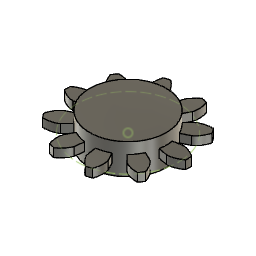
Tank Track Gear small v6 (Autodesk Fusion 360 design; units mm, degrees)
description: Spur Gear; Module: 3.0; Num Teeth: 10; Pressure Angle: 20.0; Backlash: 0.00 mm
Autodesk Fusion 360 part; units mm, degrees
(part 1 of 4)
sketch "Sketch1" plane through (0, 0, 0) normal (0, 0, 1) x (1, 0, 0) in component "Spur Gear (10 teeth)"
  circle A0 centre (0, 0) radius 11.3492
extrude "Extrude1" add sketch "Sketch1" along normal blind 2.5 in component "Spur Gear (10 teeth)"
sketch "Sketch2" plane through (0, 0, 0) normal (0, 0, 1) x (1, 0, 0) in component "Spur Gear (10 teeth)"
  spline S0 degree 5 poles (13.8874, -2.4122) (13.899, -2.4142) (13.9221, -2.4178) (13.9569, -2.422) (14.0035, -2.4254) (14.0621, -2.4264) (14.1209, -2.4253) (14.1799, -2.4228) (14.239, -2.4196) (14.2982, -2.4158) (14.3573, -2.4115) (14.4166, -2.4064) (14.4759, -2.4004) (14.5353, -2.3932) (14.5948, -2.3849) (14.6543, -2.3756) (14.7138, -2.3655) (14.7734, -2.3546) (14.8329, -2.343) (14.8925, -2.3309) (14.9521, -2.3181) (15.0117, -2.3046) (15.0713, -2.2905) (15.1308, -2.2756) (15.1904, -2.26) (15.25, -2.2438) (15.3095, -2.2269) (15.3691, -2.2094) (15.4286, -2.1913) (15.488, -2.1727) (15.5475, -2.1534) (15.6069, -2.1336) (15.6662, -2.1132) (15.7256, -2.0922) (15.7848, -2.0706) (15.8441, -2.0485) (15.9033, -2.0258) (15.9624, -2.0026) (16.0215, -1.9789) (16.0805, -1.9546) (16.1394, -1.9298) (16.1983, -1.9045) (16.2571, -1.8786) (16.3159, -1.8523) (16.3745, -1.8254) (16.4331, -1.798) (16.4917, -1.7701) (16.5501, -1.7418) (16.6085, -1.7129) (16.6667, -1.6835) (16.7249, -1.6537) (16.783, -1.6234) (16.841, -1.5926) (16.8989, -1.5613) (16.9568, -1.5296) (17.0145, -1.4974) (17.0721, -1.4647) (17.1296, -1.4316) (17.187, -1.398) (17.2443, -1.364) (17.3015, -1.3295) (17.3586, -1.2945) (17.4155, -1.2591) (17.4724, -1.2233) (17.5291, -1.187) (17.5857, -1.1503) (17.6422, -1.1132) (17.6986, -1.0756) (17.7548, -1.0376) (17.8109, -0.9992) (17.8669, -0.9603) (17.9116, -0.9289) (17.945, -0.9051) (17.9673, -0.8892) (17.9784, -0.8812) knots 0 0 0 0 0 0 0.01428571 0.02857143 0.04285714 0.05714286 0.07142857 0.08571429 0.1 0.11428571 0.12857143 0.14285714 0.15714286 0.17142857 0.18571429 0.2 0.21428571 0.22857143 0.24285714 0.25714286 0.27142857 0.28571429 0.3 0.31428571 0.32857143 0.34285714 0.35714286 0.37142857 0.38571429 0.4 0.41428571 0.42857143 0.44285714 0.45714286 0.47142857 0.48571429 0.5 0.51428571 0.52857143 0.54285714 0.55714286 0.57142857 0.58571429 0.6 0.61428571 0.62857143 0.64285714 0.65714286 0.67142857 0.68571429 0.7 0.71428571 0.72857143 0.74285714 0.75714286 0.77142857 0.78571429 0.8 0.81428571 0.82857143 0.84285714 0.85714286 0.87142857 0.88571429 0.9 0.91428571 0.92857143 0.94285714 0.95714286 0.97142857 0.98571429 1 1 1 1 1 1
  spline S1 degree 5 poles (13.8874, 2.4122) (13.899, 2.4142) (13.9221, 2.4178) (13.9569, 2.422) (14.0035, 2.4254) (14.0621, 2.4264) (14.1209, 2.4253) (14.1799, 2.4228) (14.239, 2.4196) (14.2982, 2.4158) (14.3573, 2.4115) (14.4166, 2.4064) (14.4759, 2.4004) (14.5353, 2.3932) (14.5948, 2.3849) (14.6543, 2.3756) (14.7138, 2.3655) (14.7734, 2.3546) (14.8329, 2.343) (14.8925, 2.3309) (14.9521, 2.3181) (15.0117, 2.3046) (15.0713, 2.2905) (15.1308, 2.2756) (15.1904, 2.26) (15.25, 2.2438) (15.3095, 2.2269) (15.3691, 2.2094) (15.4286, 2.1913) (15.488, 2.1727) (15.5475, 2.1534) (15.6069, 2.1336) (15.6662, 2.1132) (15.7256, 2.0922) (15.7848, 2.0706) (15.8441, 2.0485) (15.9033, 2.0258) (15.9624, 2.0026) (16.0215, 1.9789) (16.0805, 1.9546) (16.1394, 1.9298) (16.1983, 1.9045) (16.2571, 1.8786) (16.3159, 1.8523) (16.3745, 1.8254) (16.4331, 1.798) (16.4917, 1.7701) (16.5501, 1.7418) (16.6085, 1.7129) (16.6667, 1.6835) (16.7249, 1.6537) (16.783, 1.6234) (16.841, 1.5926) (16.8989, 1.5613) (16.9568, 1.5296) (17.0145, 1.4974) (17.0721, 1.4647) (17.1296, 1.4316) (17.187, 1.398) (17.2443, 1.364) (17.3015, 1.3295) (17.3586, 1.2945) (17.4155, 1.2591) (17.4724, 1.2233) (17.5291, 1.187) (17.5857, 1.1503) (17.6422, 1.1132) (17.6986, 1.0756) (17.7548, 1.0376) (17.8109, 0.9992) (17.8669, 0.9603) (17.9116, 0.9289) (17.945, 0.9051) (17.9673, 0.8892) (17.9784, 0.8812) knots 0 0 0 0 0 0 0.01428571 0.02857143 0.04285714 0.05714286 0.07142857 0.08571429 0.1 0.11428571 0.12857143 0.14285714 0.15714286 0.17142857 0.18571429 0.2 0.21428571 0.22857143 0.24285714 0.25714286 0.27142857 0.28571429 0.3 0.31428571 0.32857143 0.34285714 0.35714286 0.37142857 0.38571429 0.4 0.41428571 0.42857143 0.44285714 0.45714286 0.47142857 0.48571429 0.5 0.51428571 0.52857143 0.54285714 0.55714286 0.57142857 0.58571429 0.6 0.61428571 0.62857143 0.64285714 0.65714286 0.67142857 0.68571429 0.7 0.71428571 0.72857143 0.74285714 0.75714286 0.77142857 0.78571429 0.8 0.81428571 0.82857143 0.84285714 0.85714286 0.87142857 0.88571429 0.9 0.91428571 0.92857143 0.94285714 0.95714286 0.97142857 0.98571429 1 1 1 1 1 1
  arc A0 (17.9784, -0.8812) -> (17.9784, 0.8812) centre (0, 0) ccw
  line L0 (11.1719, -1.9423) -> (13.8874, -2.4122)
  line L1 (11.1719, 1.9423) -> (13.8874, 2.4122)
  line L2 (11.1719, -1.9423) -> (11.1719, 1.9423)
  point P0 (14.1686, -2.4231)
  point P1 (14.4549, -2.4023)
  point P2 (14.7445, -2.3598)
  point P3 (15.0363, -2.2987)
  point P4 (15.3299, -2.2208)
  point P5 (15.6246, -2.1274)
  point P6 (15.9202, -2.0191)
  point P7 (16.2161, -1.8966)
  point P8 (16.5119, -1.7602)
  point P9 (16.8074, -1.6104)
  point P10 (17.1022, -1.4473)
  point P11 (17.3958, -1.2713)
  point P12 (17.688, -1.0826)
  point P13 (14.1686, 2.4231)
  point P14 (14.4549, 2.4023)
  point P15 (14.7445, 2.3598)
  point P16 (15.0363, 2.2987)
  point P17 (15.3299, 2.2208)
  point P18 (15.6246, 2.1274)
  point P19 (15.9202, 2.0191)
  point P20 (16.2161, 1.8966)
  point P21 (16.5119, 1.7602)
  point P22 (16.8074, 1.6104)
  point P23 (17.1022, 1.4473)
  point P24 (17.3958, 1.2713)
  point P25 (17.688, 1.0826)
extrude "Extrude2" add sketch "Sketch2" along normal blind 2.5 in component "Spur Gear (10 teeth)"
pattern_circular "C-Pattern1" count 10 over 360 about axis through (0, 0, 0) along (0, 0, 1) of "Extrude2" in component "Spur Gear (10 teeth)"
sketch "Sketch3" plane through (0, 0, 0) normal (0, 0, 1) x (1, 0, 0) in component "Spur Gear (10 teeth)"
  circle A0 centre (0, 0) radius 15 construction
sketch "Sketch1 (2)" plane through (0, 0, 2.5) normal (0, 0, 1) x (-1, 0, 0)
  arc A0 (-10.1886, 4.9996) -> (-11.1815, 1.9439) centre (0, 0) ccw
  line L0 (-11.1815, 1.9439) -> (-13.8874, 2.4122)
  spline S0 degree 5 poles (-13.8874, 2.4122) (-13.899, 2.4142) (-13.9221, 2.4178) (-13.9569, 2.422) (-14.0035, 2.4254) (-14.0621, 2.4264) (-14.1209, 2.4253) (-14.1799, 2.4228) (-14.239, 2.4196) (-14.2982, 2.4158) (-14.3573, 2.4115) (-14.4166, 2.4064) (-14.4759, 2.4004) (-14.5353, 2.3932) (-14.5948, 2.3849) (-14.6543, 2.3756) (-14.7138, 2.3655) (-14.7734, 2.3546) (-14.8329, 2.343) (-14.8925, 2.3309) (-14.9521, 2.3181) (-15.0117, 2.3046) (-15.0713, 2.2905) (-15.1308, 2.2756) (-15.1904, 2.26) (-15.25, 2.2438) (-15.3095, 2.2269) (-15.3691, 2.2094) (-15.4286, 2.1913) (-15.488, 2.1727) (-15.5475, 2.1534) (-15.6069, 2.1336) (-15.6662, 2.1132) (-15.7256, 2.0922) (-15.7848, 2.0706) (-15.8441, 2.0485) (-15.9033, 2.0258) (-15.9624, 2.0026) (-16.0215, 1.9789) (-16.0805, 1.9546) (-16.1394, 1.9298) (-16.1983, 1.9045) (-16.2571, 1.8786) (-16.3159, 1.8523) (-16.3745, 1.8254) (-16.4331, 1.798) (-16.4917, 1.7701) (-16.5501, 1.7418) (-16.6085, 1.7129) (-16.6667, 1.6835) (-16.7249, 1.6537) (-16.783, 1.6234) (-16.841, 1.5926) (-16.8989, 1.5613) (-16.9568, 1.5296) (-17.0145, 1.4974) (-17.0721, 1.4647) (-17.1296, 1.4316) (-17.187, 1.398) (-17.2443, 1.364) (-17.3015, 1.3295) (-17.3586, 1.2945) (-17.4155, 1.2591) (-17.4724, 1.2233) (-17.5291, 1.187) (-17.5857, 1.1503) (-17.6422, 1.1132) (-17.6986, 1.0756) (-17.7548, 1.0376) (-17.8109, 0.9992) (-17.8669, 0.9603) (-17.9116, 0.9289) (-17.945, 0.9051) (-17.9673, 0.8892) (-17.9784, 0.8812) knots 0 0 0 0 0 0 0.01428571 0.02857143 0.04285714 0.05714286 0.07142857 0.08571429 0.1 0.11428571 0.12857143 0.14285714 0.15714286 0.17142857 0.18571429 0.2 0.21428571 0.22857143 0.24285714 0.25714286 0.27142857 0.28571429 0.3 0.31428571 0.32857143 0.34285714 0.35714286 0.37142857 0.38571429 0.4 0.41428571 0.42857143 0.44285714 0.45714286 0.47142857 0.48571429 0.5 0.51428571 0.52857143 0.54285714 0.55714286 0.57142857 0.58571429 0.6 0.61428571 0.62857143 0.64285714 0.65714286 0.67142857 0.68571429 0.7 0.71428571 0.72857143 0.74285714 0.75714286 0.77142857 0.78571429 0.8 0.81428571 0.82857143 0.84285714 0.85714286 0.87142857 0.88571429 0.9 0.91428571 0.92857143 0.94285714 0.95714286 0.97142857 0.98571429 1 1 1 1 1 1
  arc A1 (-17.9784, 0.8812) -> (-17.9784, -0.8812) centre (0, 0) ccw
  spline S1 degree 5 poles (-17.9784, -0.8812) (-17.9673, -0.8892) (-17.945, -0.9051) (-17.9116, -0.9289) (-17.8669, -0.9603) (-17.8109, -0.9992) (-17.7548, -1.0376) (-17.6986, -1.0756) (-17.6422, -1.1132) (-17.5857, -1.1503) (-17.5291, -1.187) (-17.4724, -1.2233) (-17.4155, -1.2591) (-17.3586, -1.2945) (-17.3015, -1.3295) (-17.2443, -1.364) (-17.187, -1.398) (-17.1296, -1.4316) (-17.0721, -1.4647) (-17.0145, -1.4974) (-16.9568, -1.5296) (-16.8989, -1.5613) (-16.841, -1.5926) (-16.783, -1.6234) (-16.7249, -1.6537) (-16.6667, -1.6835) (-16.6085, -1.7129) (-16.5501, -1.7418) (-16.4917, -1.7701) (-16.4331, -1.798) (-16.3745, -1.8254) (-16.3159, -1.8523) (-16.2571, -1.8786) (-16.1983, -1.9045) (-16.1394, -1.9298) (-16.0805, -1.9546) (-16.0215, -1.9789) (-15.9624, -2.0026) (-15.9033, -2.0258) (-15.8441, -2.0485) (-15.7848, -2.0706) (-15.7256, -2.0922) (-15.6662, -2.1132) (-15.6069, -2.1336) (-15.5475, -2.1534) (-15.488, -2.1727) (-15.4286, -2.1913) (-15.3691, -2.2094) (-15.3095, -2.2269) (-15.25, -2.2438) (-15.1904, -2.26) (-15.1308, -2.2756) (-15.0713, -2.2905) (-15.0117, -2.3046) (-14.9521, -2.3181) (-14.8925, -2.3309) (-14.8329, -2.343) (-14.7734, -2.3546) (-14.7138, -2.3655) (-14.6543, -2.3756) (-14.5948, -2.3849) (-14.5353, -2.3932) (-14.4759, -2.4004) (-14.4166, -2.4064) (-14.3573, -2.4115) (-14.2982, -2.4158) (-14.239, -2.4196) (-14.1799, -2.4228) (-14.1209, -2.4253) (-14.0621, -2.4264) (-14.0035, -2.4254) (-13.9569, -2.422) (-13.9221, -2.4178) (-13.899, -2.4142) (-13.8874, -2.4122) knots -1 -1 -1 -1 -1 -1 -0.98571429 -0.97142857 -0.95714286 -0.94285714 -0.92857143 -0.91428571 -0.9 -0.88571429 -0.87142857 -0.85714286 -0.84285714 -0.82857143 -0.81428571 -0.8 -0.78571429 -0.77142857 -0.75714286 -0.74285714 -0.72857143 -0.71428571 -0.7 -0.68571429 -0.67142857 -0.65714286 -0.64285714 -0.62857143 -0.61428571 -0.6 -0.58571429 -0.57142857 -0.55714286 -0.54285714 -0.52857143 -0.51428571 -0.5 -0.48571429 -0.47142857 -0.45714286 -0.44285714 -0.42857143 -0.41428571 -0.4 -0.38571429 -0.37142857 -0.35714286 -0.34285714 -0.32857143 -0.31428571 -0.3 -0.28571429 -0.27142857 -0.25714286 -0.24285714 -0.22857143 -0.21428571 -0.2 -0.18571429 -0.17142857 -0.15714286 -0.14285714 -0.12857143 -0.11428571 -0.1 -0.08571429 -0.07142857 -0.05714286 -0.04285714 -0.02857143 -0.01428571 0 0 0 0 0 0
  line L1 (-13.8874, -2.4122) -> (-11.1815, -1.9439)
  arc A2 (-11.1815, -1.9439) -> (-10.1886, -4.9996) centre (0, 0) ccw
  line L2 (-10.1886, -4.9996) -> (-12.6531, -6.2113)
  spline S2 degree 5 poles (-12.6531, -6.2113) (-12.6636, -6.2165) (-12.6844, -6.2271) (-12.715, -6.2442) (-12.7547, -6.2689) (-12.8027, -6.3025) (-12.8496, -6.338) (-12.8959, -6.3747) (-12.9418, -6.412) (-12.9874, -6.4498) (-13.0328, -6.4881) (-13.0777, -6.527) (-13.1222, -6.5668) (-13.166, -6.6075) (-13.2092, -6.6491) (-13.2519, -6.6916) (-13.2941, -6.7349) (-13.3359, -6.7787) (-13.3773, -6.823) (-13.4183, -6.8679) (-13.459, -6.9133) (-13.4993, -6.9592) (-13.5392, -7.0056) (-13.5787, -7.0527) (-13.6177, -7.1003) (-13.6564, -7.1485) (-13.6946, -7.1971) (-13.7325, -7.2463) (-13.77, -7.2959) (-13.8071, -7.3459) (-13.8439, -7.3964) (-13.8803, -7.4474) (-13.9163, -7.4988) (-13.952, -7.5506) (-13.9873, -7.6029) (-14.0222, -7.6556) (-14.0568, -7.7088) (-14.091, -7.7623) (-14.1248, -7.8162) (-14.1583, -7.8706) (-14.1914, -7.9253) (-14.2241, -7.9804) (-14.2565, -8.0359) (-14.2885, -8.0917) (-14.3202, -8.1479) (-14.3515, -8.2045) (-14.3825, -8.2615) (-14.4131, -8.3188) (-14.4433, -8.3764) (-14.4732, -8.4344) (-14.5028, -8.4928) (-14.532, -8.5515) (-14.5608, -8.6105) (-14.5893, -8.6698) (-14.6174, -8.7295) (-14.6451, -8.7894) (-14.6726, -8.8497) (-14.6996, -8.9103) (-14.7263, -8.9713) (-14.7527, -9.0325) (-14.7786, -9.094) (-14.8043, -9.1558) (-14.8296, -9.2179) (-14.8545, -9.2803) (-14.8791, -9.343) (-14.9033, -9.406) (-14.9272, -9.4692) (-14.9507, -9.5328) (-14.9738, -9.5966) (-14.9966, -9.6606) (-15.0191, -9.725) (-15.0367, -9.7767) (-15.0498, -9.8156) (-15.0585, -9.8415) (-15.0628, -9.8545) knots 0 0 0 0 0 0 0.01428571 0.02857143 0.04285714 0.05714286 0.07142857 0.08571429 0.1 0.11428571 0.12857143 0.14285714 0.15714286 0.17142857 0.18571429 0.2 0.21428571 0.22857143 0.24285714 0.25714286 0.27142857 0.28571429 0.3 0.31428571 0.32857143 0.34285714 0.35714286 0.37142857 0.38571429 0.4 0.41428571 0.42857143 0.44285714 0.45714286 0.47142857 0.48571429 0.5 0.51428571 0.52857143 0.54285714 0.55714286 0.57142857 0.58571429 0.6 0.61428571 0.62857143 0.64285714 0.65714286 0.67142857 0.68571429 0.7 0.71428571 0.72857143 0.74285714 0.75714286 0.77142857 0.78571429 0.8 0.81428571 0.82857143 0.84285714 0.85714286 0.87142857 0.88571429 0.9 0.91428571 0.92857143 0.94285714 0.95714286 0.97142857 0.98571429 1 1 1 1 1 1
  arc A3 (-15.0628, -9.8545) -> (-14.0269, -11.2804) centre (0, 0) ccw
  spline S3 degree 5 poles (-14.0269, -11.2804) (-14.0132, -11.2803) (-13.9858, -11.2801) (-13.9448, -11.2796) (-13.8902, -11.2788) (-13.822, -11.2773) (-13.754, -11.2754) (-13.6862, -11.2731) (-13.6185, -11.2704) (-13.551, -11.2673) (-13.4836, -11.2637) (-13.4164, -11.2597) (-13.3494, -11.2553) (-13.2825, -11.2504) (-13.2158, -11.2451) (-13.1492, -11.2394) (-13.0829, -11.2333) (-13.0167, -11.2267) (-12.9507, -11.2197) (-12.8849, -11.2123) (-12.8192, -11.2044) (-12.7538, -11.1961) (-12.6886, -11.1873) (-12.6235, -11.1782) (-12.5587, -11.1685) (-12.4941, -11.1585) (-12.4297, -11.148) (-12.3655, -11.137) (-12.3016, -11.1256) (-12.2378, -11.1138) (-12.1743, -11.1015) (-12.1111, -11.0887) (-12.0481, -11.0755) (-11.9853, -11.0619) (-11.9228, -11.0477) (-11.8605, -11.0332) (-11.7985, -11.0181) (-11.7367, -11.0026) (-11.6752, -10.9866) (-11.614, -10.9702) (-11.5531, -10.9533) (-11.4925, -10.9359) (-11.4322, -10.918) (-11.3721, -10.8996) (-11.3124, -10.8807) (-11.253, -10.8614) (-11.1939, -10.8415) (-11.1352, -10.8212) (-11.0767, -10.8003) (-11.0186, -10.779) (-10.9609, -10.7571) (-10.9036, -10.7347) (-10.8466, -10.7117) (-10.7901, -10.6881) (-10.734, -10.664) (-10.6782, -10.6393) (-10.6229, -10.6141) (-10.5679, -10.5884) (-10.5133, -10.5623) (-10.4592, -10.5355) (-10.4056, -10.508) (-10.3526, -10.4798) (-10.3004, -10.4507) (-10.2488, -10.4207) (-10.1979, -10.39) (-10.1475, -10.3587) (-10.0974, -10.3269) (-10.0477, -10.2948) (-9.9985, -10.2622) (-9.9503, -10.2285) (-9.9035, -10.1932) (-9.8677, -10.1631) (-9.842, -10.1393) (-9.8255, -10.1228) (-9.8173, -10.1144) knots -1 -1 -1 -1 -1 -1 -0.98571429 -0.97142857 -0.95714286 -0.94285714 -0.92857143 -0.91428571 -0.9 -0.88571429 -0.87142857 -0.85714286 -0.84285714 -0.82857143 -0.81428571 -0.8 -0.78571429 -0.77142857 -0.75714286 -0.74285714 -0.72857143 -0.71428571 -0.7 -0.68571429 -0.67142857 -0.65714286 -0.64285714 -0.62857143 -0.61428571 -0.6 -0.58571429 -0.57142857 -0.55714286 -0.54285714 -0.52857143 -0.51428571 -0.5 -0.48571429 -0.47142857 -0.45714286 -0.44285714 -0.42857143 -0.41428571 -0.4 -0.38571429 -0.37142857 -0.35714286 -0.34285714 -0.32857143 -0.31428571 -0.3 -0.28571429 -0.27142857 -0.25714286 -0.24285714 -0.22857143 -0.21428571 -0.2 -0.18571429 -0.17142857 -0.15714286 -0.14285714 -0.12857143 -0.11428571 -0.1 -0.08571429 -0.07142857 -0.05714286 -0.04285714 -0.02857143 -0.01428571 0 0 0 0 0 0
  line L3 (-9.8173, -10.1144) -> (-7.9034, -8.145)
  arc A4 (-7.9034, -8.145) -> (-5.3041, -10.0335) centre (0, 0) ccw
  line L4 (-5.3041, -10.0335) -> (-6.5856, -12.4623)
  spline S4 degree 5 poles (-6.5856, -12.4623) (-6.5911, -12.4727) (-6.6017, -12.4936) (-6.6164, -12.5253) (-6.634, -12.5687) (-6.6531, -12.6241) (-6.6702, -12.6804) (-6.6861, -12.7372) (-6.7012, -12.7944) (-6.7159, -12.8518) (-6.7301, -12.9095) (-6.7436, -12.9674) (-6.7562, -13.0257) (-6.7677, -13.0844) (-6.7782, -13.1435) (-6.7878, -13.2029) (-6.7965, -13.2627) (-6.8045, -13.3227) (-6.812, -13.3829) (-6.8188, -13.4433) (-6.8251, -13.504) (-6.8307, -13.5648) (-6.8356, -13.6258) (-6.8399, -13.6871) (-6.8435, -13.7486) (-6.8465, -13.8102) (-6.8488, -13.8721) (-6.8506, -13.9341) (-6.8518, -13.9963) (-6.8524, -14.0586) (-6.8524, -14.1211) (-6.852, -14.1837) (-6.8509, -14.2465) (-6.8493, -14.3094) (-6.8471, -14.3724) (-6.8443, -14.4356) (-6.8411, -14.4989) (-6.8373, -14.5623) (-6.8329, -14.6258) (-6.8281, -14.6894) (-6.8227, -14.7532) (-6.8168, -14.817) (-6.8104, -14.8809) (-6.8035, -14.9449) (-6.7961, -15.009) (-6.7881, -15.0732) (-6.7797, -15.1375) (-6.7708, -15.2019) (-6.7614, -15.2663) (-6.7515, -15.3308) (-6.7411, -15.3953) (-6.7302, -15.4599) (-6.7188, -15.5246) (-6.707, -15.5894) (-6.6947, -15.6542) (-6.6819, -15.719) (-6.6686, -15.7839) (-6.6549, -15.8488) (-6.6407, -15.9138) (-6.626, -15.9788) (-6.6109, -16.0439) (-6.5953, -16.109) (-6.5792, -16.1741) (-6.5627, -16.2392) (-6.5457, -16.3044) (-6.5283, -16.3695) (-6.5104, -16.4347) (-6.4921, -16.5) (-6.4734, -16.5652) (-6.4541, -16.6304) (-6.4345, -16.6957) (-6.4184, -16.7479) (-6.4061, -16.787) (-6.3979, -16.8131) (-6.3937, -16.8262) knots 0 0 0 0 0 0 0.01428571 0.02857143 0.04285714 0.05714286 0.07142857 0.08571429 0.1 0.11428571 0.12857143 0.14285714 0.15714286 0.17142857 0.18571429 0.2 0.21428571 0.22857143 0.24285714 0.25714286 0.27142857 0.28571429 0.3 0.31428571 0.32857143 0.34285714 0.35714286 0.37142857 0.38571429 0.4 0.41428571 0.42857143 0.44285714 0.45714286 0.47142857 0.48571429 0.5 0.51428571 0.52857143 0.54285714 0.55714286 0.57142857 0.58571429 0.6 0.61428571 0.62857143 0.64285714 0.65714286 0.67142857 0.68571429 0.7 0.71428571 0.72857143 0.74285714 0.75714286 0.77142857 0.78571429 0.8 0.81428571 0.82857143 0.84285714 0.85714286 0.87142857 0.88571429 0.9 0.91428571 0.92857143 0.94285714 0.95714286 0.97142857 0.98571429 1 1 1 1 1 1
  arc A5 (-6.3937, -16.8262) -> (-4.7175, -17.3708) centre (0, 0) ccw
  spline S5 degree 5 poles (-4.7175, -17.3708) (-4.7065, -17.3627) (-4.6845, -17.3464) (-4.6516, -17.3219) (-4.6079, -17.2892) (-4.5536, -17.2479) (-4.4997, -17.2065) (-4.4462, -17.1647) (-4.393, -17.1227) (-4.3403, -17.0805) (-4.2879, -17.038) (-4.2358, -16.9952) (-4.1842, -16.9523) (-4.1329, -16.909) (-4.0821, -16.8655) (-4.0316, -16.8218) (-3.9815, -16.7778) (-3.9318, -16.7336) (-3.8825, -16.6891) (-3.8337, -16.6444) (-3.7852, -16.5995) (-3.7371, -16.5543) (-3.6895, -16.5089) (-3.6423, -16.4633) (-3.5955, -16.4174) (-3.5492, -16.3713) (-3.5032, -16.3249) (-3.4578, -16.2783) (-3.4127, -16.2315) (-3.3681, -16.1845) (-3.324, -16.1372) (-3.2803, -16.0897) (-3.2371, -16.042) (-3.1943, -15.994) (-3.152, -15.9458) (-3.1102, -15.8974) (-3.0689, -15.8488) (-3.028, -15.8) (-2.9877, -15.7509) (-2.9478, -15.7016) (-2.9085, -15.6521) (-2.8697, -15.6024) (-2.8314, -15.5525) (-2.7936, -15.5023) (-2.7564, -15.452) (-2.7197, -15.4014) (-2.6836, -15.3506) (-2.648, -15.2996) (-2.613, -15.2484) (-2.5785, -15.197) (-2.5447, -15.1453) (-2.5115, -15.0935) (-2.4789, -15.0414) (-2.447, -14.9891) (-2.4158, -14.9366) (-2.3853, -14.8839) (-2.3553, -14.831) (-2.3259, -14.7779) (-2.2971, -14.7246) (-2.2691, -14.6711) (-2.2418, -14.6174) (-2.2156, -14.5634) (-2.1904, -14.5092) (-2.1664, -14.4546) (-2.1432, -14.3998) (-2.1208, -14.3449) (-2.099, -14.2898) (-2.0776, -14.2346) (-2.057, -14.1793) (-2.0378, -14.1237) (-2.0207, -14.0676) (-2.0094, -14.0223) (-2.0027, -13.9879) (-1.9989, -13.9648) (-1.9973, -13.9532) knots -1 -1 -1 -1 -1 -1 -0.98571429 -0.97142857 -0.95714286 -0.94285714 -0.92857143 -0.91428571 -0.9 -0.88571429 -0.87142857 -0.85714286 -0.84285714 -0.82857143 -0.81428571 -0.8 -0.78571429 -0.77142857 -0.75714286 -0.74285714 -0.72857143 -0.71428571 -0.7 -0.68571429 -0.67142857 -0.65714286 -0.64285714 -0.62857143 -0.61428571 -0.6 -0.58571429 -0.57142857 -0.55714286 -0.54285714 -0.52857143 -0.51428571 -0.5 -0.48571429 -0.47142857 -0.45714286 -0.44285714 -0.42857143 -0.41428571 -0.4 -0.38571429 -0.37142857 -0.35714286 -0.34285714 -0.32857143 -0.31428571 -0.3 -0.28571429 -0.27142857 -0.25714286 -0.24285714 -0.22857143 -0.21428571 -0.2 -0.18571429 -0.17142857 -0.15714286 -0.14285714 -0.12857143 -0.11428571 -0.1 -0.08571429 -0.07142857 -0.05714286 -0.04285714 -0.02857143 -0.01428571 0 0 0 0 0 0
  line L5 (-1.9973, -13.9532) -> (-1.6065, -11.2349)
  arc A6 (-1.6065, -11.2349) -> (1.6065, -11.2349) centre (0, 0) ccw
  line L6 (1.6065, -11.2349) -> (1.9973, -13.9532)
  spline S6 degree 5 poles (1.9973, -13.9532) (1.9989, -13.9648) (2.0027, -13.9879) (2.0094, -14.0223) (2.0207, -14.0676) (2.0378, -14.1237) (2.057, -14.1793) (2.0776, -14.2346) (2.099, -14.2898) (2.1208, -14.3449) (2.1432, -14.3998) (2.1664, -14.4546) (2.1904, -14.5092) (2.2156, -14.5634) (2.2418, -14.6174) (2.2691, -14.6711) (2.2971, -14.7246) (2.3259, -14.7779) (2.3553, -14.831) (2.3853, -14.8839) (2.4158, -14.9366) (2.447, -14.9891) (2.4789, -15.0414) (2.5115, -15.0935) (2.5447, -15.1453) (2.5785, -15.197) (2.613, -15.2484) (2.648, -15.2996) (2.6836, -15.3506) (2.7197, -15.4014) (2.7564, -15.452) (2.7936, -15.5023) (2.8314, -15.5525) (2.8697, -15.6024) (2.9085, -15.6521) (2.9478, -15.7016) (2.9877, -15.7509) (3.028, -15.8) (3.0689, -15.8488) (3.1102, -15.8974) (3.152, -15.9458) (3.1943, -15.994) (3.2371, -16.042) (3.2803, -16.0897) (3.324, -16.1372) (3.3681, -16.1845) (3.4127, -16.2315) (3.4578, -16.2783) (3.5032, -16.3249) (3.5492, -16.3713) (3.5955, -16.4174) (3.6423, -16.4633) (3.6895, -16.5089) (3.7371, -16.5543) (3.7852, -16.5995) (3.8337, -16.6444) (3.8825, -16.6891) (3.9318, -16.7336) (3.9815, -16.7778) (4.0316, -16.8218) (4.0821, -16.8655) (4.1329, -16.909) (4.1842, -16.9523) (4.2358, -16.9952) (4.2879, -17.038) (4.3403, -17.0805) (4.393, -17.1227) (4.4462, -17.1647) (4.4997, -17.2065) (4.5536, -17.2479) (4.6079, -17.2892) (4.6516, -17.3219) (4.6845, -17.3464) (4.7065, -17.3627) (4.7175, -17.3708) knots 0 0 0 0 0 0 0.01428571 0.02857143 0.04285714 0.05714286 0.07142857 0.08571429 0.1 0.11428571 0.12857143 0.14285714 0.15714286 0.17142857 0.18571429 0.2 0.21428571 0.22857143 0.24285714 0.25714286 0.27142857 0.28571429 0.3 0.31428571 0.32857143 0.34285714 0.35714286 0.37142857 0.38571429 0.4 0.41428571 0.42857143 0.44285714 0.45714286 0.47142857 0.48571429 0.5 0.51428571 0.52857143 0.54285714 0.55714286 0.57142857 0.58571429 0.6 0.61428571 0.62857143 0.64285714 0.65714286 0.67142857 0.68571429 0.7 0.71428571 0.72857143 0.74285714 0.75714286 0.77142857 0.78571429 0.8 0.81428571 0.82857143 0.84285714 0.85714286 0.87142857 0.88571429 0.9 0.91428571 0.92857143 0.94285714 0.95714286 0.97142857 0.98571429 1 1 1 1 1 1
  arc A7 (4.7175, -17.3708) -> (6.3937, -16.8262) centre (0, 0) ccw
  spline S7 degree 5 poles (6.3937, -16.8262) (6.3979, -16.8131) (6.4061, -16.787) (6.4184, -16.7479) (6.4345, -16.6957) (6.4541, -16.6304) (6.4734, -16.5652) (6.4921, -16.5) (6.5104, -16.4347) (6.5283, -16.3695) (6.5457, -16.3044) (6.5627, -16.2392) (6.5792, -16.1741) (6.5953, -16.109) (6.6109, -16.0439) (6.626, -15.9788) (6.6407, -15.9138) (6.6549, -15.8488) (6.6686, -15.7839) (6.6819, -15.719) (6.6947, -15.6542) (6.707, -15.5894) (6.7188, -15.5246) (6.7302, -15.4599) (6.7411, -15.3953) (6.7515, -15.3308) (6.7614, -15.2663) (6.7708, -15.2019) (6.7797, -15.1375) (6.7881, -15.0732) (6.7961, -15.009) (6.8035, -14.9449) (6.8104, -14.8809) (6.8168, -14.817) (6.8227, -14.7532) (6.8281, -14.6894) (6.8329, -14.6258) (6.8373, -14.5623) (6.8411, -14.4989) (6.8443, -14.4356) (6.8471, -14.3724) (6.8493, -14.3094) (6.8509, -14.2465) (6.852, -14.1837) (6.8524, -14.1211) (6.8524, -14.0586) (6.8518, -13.9963) (6.8506, -13.9341) (6.8488, -13.8721) (6.8465, -13.8102) (6.8435, -13.7486) (6.8399, -13.6871) (6.8356, -13.6258) (6.8307, -13.5648) (6.8251, -13.504) (6.8188, -13.4433) (6.812, -13.3829) (6.8045, -13.3227) (6.7965, -13.2627) (6.7878, -13.2029) (6.7782, -13.1435) (6.7677, -13.0844) (6.7562, -13.0257) (6.7436, -12.9674) (6.7301, -12.9095) (6.7159, -12.8518) (6.7012, -12.7944) (6.6861, -12.7372) (6.6702, -12.6804) (6.6531, -12.6241) (6.634, -12.5687) (6.6164, -12.5253) (6.6017, -12.4936) (6.5911, -12.4727) (6.5856, -12.4623) knots -1 -1 -1 -1 -1 -1 -0.98571429 -0.97142857 -0.95714286 -0.94285714 -0.92857143 -0.91428571 -0.9 -0.88571429 -0.87142857 -0.85714286 -0.84285714 -0.82857143 -0.81428571 -0.8 -0.78571429 -0.77142857 -0.75714286 -0.74285714 -0.72857143 -0.71428571 -0.7 -0.68571429 -0.67142857 -0.65714286 -0.64285714 -0.62857143 -0.61428571 -0.6 -0.58571429 -0.57142857 -0.55714286 -0.54285714 -0.52857143 -0.51428571 -0.5 -0.48571429 -0.47142857 -0.45714286 -0.44285714 -0.42857143 -0.41428571 -0.4 -0.38571429 -0.37142857 -0.35714286 -0.34285714 -0.32857143 -0.31428571 -0.3 -0.28571429 -0.27142857 -0.25714286 -0.24285714 -0.22857143 -0.21428571 -0.2 -0.18571429 -0.17142857 -0.15714286 -0.14285714 -0.12857143 -0.11428571 -0.1 -0.08571429 -0.07142857 -0.05714286 -0.04285714 -0.02857143 -0.01428571 0 0 0 0 0 0
  line L7 (6.5856, -12.4623) -> (5.3041, -10.0335)
  arc A8 (5.3041, -10.0335) -> (7.9034, -8.145) centre (0, 0) ccw
  line L8 (7.9034, -8.145) -> (9.8173, -10.1144)
  spline S8 degree 5 poles (9.8173, -10.1144) (9.8255, -10.1228) (9.842, -10.1393) (9.8677, -10.1631) (9.9035, -10.1932) (9.9503, -10.2285) (9.9985, -10.2622) (10.0477, -10.2948) (10.0974, -10.3269) (10.1475, -10.3587) (10.1979, -10.39) (10.2488, -10.4207) (10.3004, -10.4507) (10.3526, -10.4798) (10.4056, -10.508) (10.4592, -10.5355) (10.5133, -10.5623) (10.5679, -10.5884) (10.6229, -10.6141) (10.6782, -10.6393) (10.734, -10.664) (10.7901, -10.6881) (10.8466, -10.7117) (10.9036, -10.7347) (10.9609, -10.7571) (11.0186, -10.779) (11.0767, -10.8003) (11.1352, -10.8212) (11.1939, -10.8415) (11.253, -10.8614) (11.3124, -10.8807) (11.3721, -10.8996) (11.4322, -10.918) (11.4925, -10.9359) (11.5531, -10.9533) (11.614, -10.9702) (11.6752, -10.9866) (11.7367, -11.0026) (11.7985, -11.0181) (11.8605, -11.0332) (11.9228, -11.0477) (11.9853, -11.0619) (12.0481, -11.0755) (12.1111, -11.0887) (12.1743, -11.1015) (12.2378, -11.1138) (12.3016, -11.1256) (12.3655, -11.137) (12.4297, -11.148) (12.4941, -11.1585) (12.5587, -11.1685) (12.6235, -11.1782) (12.6886, -11.1873) (12.7538, -11.1961) (12.8192, -11.2044) (12.8849, -11.2123) (12.9507, -11.2197) (13.0167, -11.2267) (13.0829, -11.2333) (13.1492, -11.2394) (13.2158, -11.2451) (13.2825, -11.2504) (13.3494, -11.2553) (13.4164, -11.2597) (13.4836, -11.2637) (13.551, -11.2673) (13.6185, -11.2704) (13.6862, -11.2731) (13.754, -11.2754) (13.822, -11.2773) (13.8902, -11.2788) (13.9448, -11.2796) (13.9858, -11.2801) (14.0132, -11.2803) (14.0269, -11.2804) knots 0 0 0 0 0 0 0.01428571 0.02857143 0.04285714 0.05714286 0.07142857 0.08571429 0.1 0.11428571 0.12857143 0.14285714 0.15714286 0.17142857 0.18571429 0.2 0.21428571 0.22857143 0.24285714 0.25714286 0.27142857 0.28571429 0.3 0.31428571 0.32857143 0.34285714 0.35714286 0.37142857 0.38571429 0.4 0.41428571 0.42857143 0.44285714 0.45714286 0.47142857 0.48571429 0.5 0.51428571 0.52857143 0.54285714 0.55714286 0.57142857 0.58571429 0.6 0.61428571 0.62857143 0.64285714 0.65714286 0.67142857 0.68571429 0.7 0.71428571 0.72857143 0.74285714 0.75714286 0.77142857 0.78571429 0.8 0.81428571 0.82857143 0.84285714 0.85714286 0.87142857 0.88571429 0.9 0.91428571 0.92857143 0.94285714 0.95714286 0.97142857 0.98571429 1 1 1 1 1 1
  arc A9 (14.0269, -11.2804) -> (15.0628, -9.8545) centre (0, 0) ccw
  spline S9 degree 5 poles (15.0628, -9.8545) (15.0585, -9.8415) (15.0498, -9.8156) (15.0367, -9.7767) (15.0191, -9.725) (14.9966, -9.6606) (14.9738, -9.5966) (14.9507, -9.5328) (14.9272, -9.4692) (14.9033, -9.406) (14.8791, -9.343) (14.8545, -9.2803) (14.8296, -9.2179) (14.8043, -9.1558) (14.7786, -9.094) (14.7527, -9.0325) (14.7263, -8.9713) (14.6996, -8.9103) (14.6726, -8.8497) (14.6451, -8.7894) (14.6174, -8.7295) (14.5893, -8.6698) (14.5608, -8.6105) (14.532, -8.5515) (14.5028, -8.4928) (14.4732, -8.4344) (14.4433, -8.3764) (14.4131, -8.3188) (14.3825, -8.2615) (14.3515, -8.2045) (14.3202, -8.1479) (14.2885, -8.0917) (14.2565, -8.0359) (14.2241, -7.9804) (14.1914, -7.9253) (14.1583, -7.8706) (14.1248, -7.8162) (14.091, -7.7623) (14.0568, -7.7088) (14.0222, -7.6556) (13.9873, -7.6029) (13.952, -7.5506) (13.9163, -7.4988) (13.8803, -7.4474) (13.8439, -7.3964) (13.8071, -7.3459) (13.77, -7.2959) (13.7325, -7.2463) (13.6946, -7.1971) (13.6564, -7.1485) (13.6177, -7.1003) (13.5787, -7.0527) (13.5392, -7.0056) (13.4993, -6.9592) (13.459, -6.9133) (13.4183, -6.8679) (13.3773, -6.823) (13.3359, -6.7787) (13.2941, -6.7349) (13.2519, -6.6916) (13.2092, -6.6491) (13.166, -6.6075) (13.1222, -6.5668) (13.0777, -6.527) (13.0328, -6.4881) (12.9874, -6.4498) (12.9418, -6.412) (12.8959, -6.3747) (12.8496, -6.338) (12.8027, -6.3025) (12.7547, -6.2689) (12.715, -6.2442) (12.6844, -6.2271) (12.6636, -6.2165) (12.6531, -6.2113) knots -1 -1 -1 -1 -1 -1 -0.98571429 -0.97142857 -0.95714286 -0.94285714 -0.92857143 -0.91428571 -0.9 -0.88571429 -0.87142857 -0.85714286 -0.84285714 -0.82857143 -0.81428571 -0.8 -0.78571429 -0.77142857 -0.75714286 -0.74285714 -0.72857143 -0.71428571 -0.7 -0.68571429 -0.67142857 -0.65714286 -0.64285714 -0.62857143 -0.61428571 -0.6 -0.58571429 -0.57142857 -0.55714286 -0.54285714 -0.52857143 -0.51428571 -0.5 -0.48571429 -0.47142857 -0.45714286 -0.44285714 -0.42857143 -0.41428571 -0.4 -0.38571429 -0.37142857 -0.35714286 -0.34285714 -0.32857143 -0.31428571 -0.3 -0.28571429 -0.27142857 -0.25714286 -0.24285714 -0.22857143 -0.21428571 -0.2 -0.18571429 -0.17142857 -0.15714286 -0.14285714 -0.12857143 -0.11428571 -0.1 -0.08571429 -0.07142857 -0.05714286 -0.04285714 -0.02857143 -0.01428571 0 0 0 0 0 0
  line L9 (12.6531, -6.2113) -> (10.1886, -4.9996)
  arc A10 (10.1886, -4.9996) -> (11.1815, -1.9439) centre (0, 0) ccw
  line L10 (11.1815, -1.9439) -> (13.8874, -2.4122)
  spline S10 degree 5 poles (13.8874, -2.4122) (13.899, -2.4142) (13.9221, -2.4178) (13.9569, -2.422) (14.0035, -2.4254) (14.0621, -2.4264) (14.1209, -2.4253) (14.1799, -2.4228) (14.239, -2.4196) (14.2982, -2.4158) (14.3573, -2.4115) (14.4166, -2.4064) (14.4759, -2.4004) (14.5353, -2.3932) (14.5948, -2.3849) (14.6543, -2.3756) (14.7138, -2.3655) (14.7734, -2.3546) (14.8329, -2.343) (14.8925, -2.3309) (14.9521, -2.3181) (15.0117, -2.3046) (15.0713, -2.2905) (15.1308, -2.2756) (15.1904, -2.26) (15.25, -2.2438) (15.3095, -2.2269) (15.3691, -2.2094) (15.4286, -2.1913) (15.488, -2.1727) (15.5475, -2.1534) (15.6069, -2.1336) (15.6662, -2.1132) (15.7256, -2.0922) (15.7848, -2.0706) (15.8441, -2.0485) (15.9033, -2.0258) (15.9624, -2.0026) (16.0215, -1.9789) (16.0805, -1.9546) (16.1394, -1.9298) (16.1983, -1.9045) (16.2571, -1.8786) (16.3159, -1.8523) (16.3745, -1.8254) (16.4331, -1.798) (16.4917, -1.7701) (16.5501, -1.7418) (16.6085, -1.7129) (16.6667, -1.6835) (16.7249, -1.6537) (16.783, -1.6234) (16.841, -1.5926) (16.8989, -1.5613) (16.9568, -1.5296) (17.0145, -1.4974) (17.0721, -1.4647) (17.1296, -1.4316) (17.187, -1.398) (17.2443, -1.364) (17.3015, -1.3295) (17.3586, -1.2945) (17.4155, -1.2591) (17.4724, -1.2233) (17.5291, -1.187) (17.5857, -1.1503) (17.6422, -1.1132) (17.6986, -1.0756) (17.7548, -1.0376) (17.8109, -0.9992) (17.8669, -0.9603) (17.9116, -0.9289) (17.945, -0.9051) (17.9673, -0.8892) (17.9784, -0.8812) knots 0 0 0 0 0 0 0.01428571 0.02857143 0.04285714 0.05714286 0.07142857 0.08571429 0.1 0.11428571 0.12857143 0.14285714 0.15714286 0.17142857 0.18571429 0.2 0.21428571 0.22857143 0.24285714 0.25714286 0.27142857 0.28571429 0.3 0.31428571 0.32857143 0.34285714 0.35714286 0.37142857 0.38571429 0.4 0.41428571 0.42857143 0.44285714 0.45714286 0.47142857 0.48571429 0.5 0.51428571 0.52857143 0.54285714 0.55714286 0.57142857 0.58571429 0.6 0.61428571 0.62857143 0.64285714 0.65714286 0.67142857 0.68571429 0.7 0.71428571 0.72857143 0.74285714 0.75714286 0.77142857 0.78571429 0.8 0.81428571 0.82857143 0.84285714 0.85714286 0.87142857 0.88571429 0.9 0.91428571 0.92857143 0.94285714 0.95714286 0.97142857 0.98571429 1 1 1 1 1 1
  arc A11 (17.9784, -0.8812) -> (17.9784, 0.8812) centre (0, 0) ccw
  spline S11 degree 5 poles (17.9784, 0.8812) (17.9673, 0.8892) (17.945, 0.9051) (17.9116, 0.9289) (17.8669, 0.9603) (17.8109, 0.9992) (17.7548, 1.0376) (17.6986, 1.0756) (17.6422, 1.1132) (17.5857, 1.1503) (17.5291, 1.187) (17.4724, 1.2233) (17.4155, 1.2591) (17.3586, 1.2945) (17.3015, 1.3295) (17.2443, 1.364) (17.187, 1.398) (17.1296, 1.4316) (17.0721, 1.4647) (17.0145, 1.4974) (16.9568, 1.5296) (16.8989, 1.5613) (16.841, 1.5926) (16.783, 1.6234) (16.7249, 1.6537) (16.6667, 1.6835) (16.6085, 1.7129) (16.5501, 1.7418) (16.4917, 1.7701) (16.4331, 1.798) (16.3745, 1.8254) (16.3159, 1.8523) (16.2571, 1.8786) (16.1983, 1.9045) (16.1394, 1.9298) (16.0805, 1.9546) (16.0215, 1.9789) (15.9624, 2.0026) (15.9033, 2.0258) (15.8441, 2.0485) (15.7848, 2.0706) (15.7256, 2.0922) (15.6662, 2.1132) (15.6069, 2.1336) (15.5475, 2.1534) (15.488, 2.1727) (15.4286, 2.1913) (15.3691, 2.2094) (15.3095, 2.2269) (15.25, 2.2438) (15.1904, 2.26) (15.1308, 2.2756) (15.0713, 2.2905) (15.0117, 2.3046) (14.9521, 2.3181) (14.8925, 2.3309) (14.8329, 2.343) (14.7734, 2.3546) (14.7138, 2.3655) (14.6543, 2.3756) (14.5948, 2.3849) (14.5353, 2.3932) (14.4759, 2.4004) (14.4166, 2.4064) (14.3573, 2.4115) (14.2982, 2.4158) (14.239, 2.4196) (14.1799, 2.4228) (14.1209, 2.4253) (14.0621, 2.4264) (14.0035, 2.4254) (13.9569, 2.422) (13.9221, 2.4178) (13.899, 2.4142) (13.8874, 2.4122) knots -1 -1 -1 -1 -1 -1 -0.98571429 -0.97142857 -0.95714286 -0.94285714 -0.92857143 -0.91428571 -0.9 -0.88571429 -0.87142857 -0.85714286 -0.84285714 -0.82857143 -0.81428571 -0.8 -0.78571429 -0.77142857 -0.75714286 -0.74285714 -0.72857143 -0.71428571 -0.7 -0.68571429 -0.67142857 -0.65714286 -0.64285714 -0.62857143 -0.61428571 -0.6 -0.58571429 -0.57142857 -0.55714286 -0.54285714 -0.52857143 -0.51428571 -0.5 -0.48571429 -0.47142857 -0.45714286 -0.44285714 -0.42857143 -0.41428571 -0.4 -0.38571429 -0.37142857 -0.35714286 -0.34285714 -0.32857143 -0.31428571 -0.3 -0.28571429 -0.27142857 -0.25714286 -0.24285714 -0.22857143 -0.21428571 -0.2 -0.18571429 -0.17142857 -0.15714286 -0.14285714 -0.12857143 -0.11428571 -0.1 -0.08571429 -0.07142857 -0.05714286 -0.04285714 -0.02857143 -0.01428571 0 0 0 0 0 0
  line L11 (13.8874, 2.4122) -> (11.1815, 1.9439)
  arc A12 (11.1815, 1.9439) -> (10.1886, 4.9996) centre (0, 0) ccw
  line L12 (10.1886, 4.9996) -> (12.6531, 6.2113)
  spline S12 degree 5 poles (12.6531, 6.2113) (12.6636, 6.2165) (12.6844, 6.2271) (12.715, 6.2442) (12.7547, 6.2689) (12.8027, 6.3025) (12.8496, 6.338) (12.8959, 6.3747) (12.9418, 6.412) (12.9874, 6.4498) (13.0328, 6.4881) (13.0777, 6.527) (13.1222, 6.5668) (13.166, 6.6075) (13.2092, 6.6491) (13.2519, 6.6916) (13.2941, 6.7349) (13.3359, 6.7787) (13.3773, 6.823) (13.4183, 6.8679) (13.459, 6.9133) (13.4993, 6.9592) (13.5392, 7.0056) (13.5787, 7.0527) (13.6177, 7.1003) (13.6564, 7.1485) (13.6946, 7.1971) (13.7325, 7.2463) (13.77, 7.2959) (13.8071, 7.3459) (13.8439, 7.3964) (13.8803, 7.4474) (13.9163, 7.4988) (13.952, 7.5506) (13.9873, 7.6029) (14.0222, 7.6556) (14.0568, 7.7088) (14.091, 7.7623) (14.1248, 7.8162) (14.1583, 7.8706) (14.1914, 7.9253) (14.2241, 7.9804) (14.2565, 8.0359) (14.2885, 8.0917) (14.3202, 8.1479) (14.3515, 8.2045) (14.3825, 8.2615) (14.4131, 8.3188) (14.4433, 8.3764) (14.4732, 8.4344) (14.5028, 8.4928) (14.532, 8.5515) (14.5608, 8.6105) (14.5893, 8.6698) (14.6174, 8.7295) (14.6451, 8.7894) (14.6726, 8.8497) (14.6996, 8.9103) (14.7263, 8.9713) (14.7527, 9.0325) (14.7786, 9.094) (14.8043, 9.1558) (14.8296, 9.2179) (14.8545, 9.2803) (14.8791, 9.343) (14.9033, 9.406) (14.9272, 9.4692) (14.9507, 9.5328) (14.9738, 9.5966) (14.9966, 9.6606) (15.0191, 9.725) (15.0367, 9.7767) (15.0498, 9.8156) (15.0585, 9.8415) (15.0628, 9.8545) knots 0 0 0 0 0 0 0.01428571 0.02857143 0.04285714 0.05714286 0.07142857 0.08571429 0.1 0.11428571 0.12857143 0.14285714 0.15714286 0.17142857 0.18571429 0.2 0.21428571 0.22857143 0.24285714 0.25714286 0.27142857 0.28571429 0.3 0.31428571 0.32857143 0.34285714 0.35714286 0.37142857 0.38571429 0.4 0.41428571 0.42857143 0.44285714 0.45714286 0.47142857 0.48571429 0.5 0.51428571 0.52857143 0.54285714 0.55714286 0.57142857 0.58571429 0.6 0.61428571 0.62857143 0.64285714 0.65714286 0.67142857 0.68571429 0.7 0.71428571 0.72857143 0.74285714 0.75714286 0.77142857 0.78571429 0.8 0.81428571 0.82857143 0.84285714 0.85714286 0.87142857 0.88571429 0.9 0.91428571 0.92857143 0.94285714 0.95714286 0.97142857 0.98571429 1 1 1 1 1 1
  arc A13 (15.0628, 9.8545) -> (14.0269, 11.2804) centre (0, 0) ccw
  spline S13 degree 5 poles (14.0269, 11.2804) (14.0132, 11.2803) (13.9858, 11.2801) (13.9448, 11.2796) (13.8902, 11.2788) (13.822, 11.2773) (13.754, 11.2754) (13.6862, 11.2731) (13.6185, 11.2704) (13.551, 11.2673) (13.4836, 11.2637) (13.4164, 11.2597) (13.3494, 11.2553) (13.2825, 11.2504) (13.2158, 11.2451) (13.1492, 11.2394) (13.0829, 11.2333) (13.0167, 11.2267) (12.9507, 11.2197) (12.8849, 11.2123) (12.8192, 11.2044) (12.7538, 11.1961) (12.6886, 11.1873) (12.6235, 11.1782) (12.5587, 11.1685) (12.4941, 11.1585) (12.4297, 11.148) (12.3655, 11.137) (12.3016, 11.1256) (12.2378, 11.1138) (12.1743, 11.1015) (12.1111, 11.0887) (12.0481, 11.0755) (11.9853, 11.0619) (11.9228, 11.0477) (11.8605, 11.0332) (11.7985, 11.0181) (11.7367, 11.0026) (11.6752, 10.9866) (11.614, 10.9702) (11.5531, 10.9533) (11.4925, 10.9359) (11.4322, 10.918) (11.3721, 10.8996) (11.3124, 10.8807) (11.253, 10.8614) (11.1939, 10.8415) (11.1352, 10.8212) (11.0767, 10.8003) (11.0186, 10.779) (10.9609, 10.7571) (10.9036, 10.7347) (10.8466, 10.7117) (10.7901, 10.6881) (10.734, 10.664) (10.6782, 10.6393) (10.6229, 10.6141) (10.5679, 10.5884) (10.5133, 10.5623) (10.4592, 10.5355) (10.4056, 10.508) (10.3526, 10.4798) (10.3004, 10.4507) (10.2488, 10.4207) (10.1979, 10.39) (10.1475, 10.3587) (10.0974, 10.3269) (10.0477, 10.2948) (9.9985, 10.2622) (9.9503, 10.2285) (9.9035, 10.1932) (9.8677, 10.1631) (9.842, 10.1393) (9.8255, 10.1228) (9.8173, 10.1144) knots -1 -1 -1 -1 -1 -1 -0.98571429 -0.97142857 -0.95714286 -0.94285714 -0.92857143 -0.91428571 -0.9 -0.88571429 -0.87142857 -0.85714286 -0.84285714 -0.82857143 -0.81428571 -0.8 -0.78571429 -0.77142857 -0.75714286 -0.74285714 -0.72857143 -0.71428571 -0.7 -0.68571429 -0.67142857 -0.65714286 -0.64285714 -0.62857143 -0.61428571 -0.6 -0.58571429 -0.57142857 -0.55714286 -0.54285714 -0.52857143 -0.51428571 -0.5 -0.48571429 -0.47142857 -0.45714286 -0.44285714 -0.42857143 -0.41428571 -0.4 -0.38571429 -0.37142857 -0.35714286 -0.34285714 -0.32857143 -0.31428571 -0.3 -0.28571429 -0.27142857 -0.25714286 -0.24285714 -0.22857143 -0.21428571 -0.2 -0.18571429 -0.17142857 -0.15714286 -0.14285714 -0.12857143 -0.11428571 -0.1 -0.08571429 -0.07142857 -0.05714286 -0.04285714 -0.02857143 -0.01428571 0 0 0 0 0 0
  line L13 (9.8173, 10.1144) -> (7.9034, 8.145)
  arc A14 (7.9034, 8.145) -> (5.3041, 10.0335) centre (0, 0) ccw
  line L14 (5.3041, 10.0335) -> (6.5856, 12.4623)
  spline S14 degree 5 poles (6.5856, 12.4623) (6.5911, 12.4727) (6.6017, 12.4936) (6.6164, 12.5253) (6.634, 12.5687) (6.6531, 12.6241) (6.6702, 12.6804) (6.6861, 12.7372) (6.7012, 12.7944) (6.7159, 12.8518) (6.7301, 12.9095) (6.7436, 12.9674) (6.7562, 13.0257) (6.7677, 13.0844) (6.7782, 13.1435) (6.7878, 13.2029) (6.7965, 13.2627) (6.8045, 13.3227) (6.812, 13.3829) (6.8188, 13.4433) (6.8251, 13.504) (6.8307, 13.5648) (6.8356, 13.6258) (6.8399, 13.6871) (6.8435, 13.7486) (6.8465, 13.8102) (6.8488, 13.8721) (6.8506, 13.9341) (6.8518, 13.9963) (6.8524, 14.0586) (6.8524, 14.1211) (6.852, 14.1837) (6.8509, 14.2465) (6.8493, 14.3094) (6.8471, 14.3724) (6.8443, 14.4356) (6.8411, 14.4989) (6.8373, 14.5623) (6.8329, 14.6258) (6.8281, 14.6894) (6.8227, 14.7532) (6.8168, 14.817) (6.8104, 14.8809) (6.8035, 14.9449) (6.7961, 15.009) (6.7881, 15.0732) (6.7797, 15.1375) (6.7708, 15.2019) (6.7614, 15.2663) (6.7515, 15.3308) (6.7411, 15.3953) (6.7302, 15.4599) (6.7188, 15.5246) (6.707, 15.5894) (6.6947, 15.6542) (6.6819, 15.719) (6.6686, 15.7839) (6.6549, 15.8488) (6.6407, 15.9138) (6.626, 15.9788) (6.6109, 16.0439) (6.5953, 16.109) (6.5792, 16.1741) (6.5627, 16.2392) (6.5457, 16.3044) (6.5283, 16.3695) (6.5104, 16.4347) (6.4921, 16.5) (6.4734, 16.5652) (6.4541, 16.6304) (6.4345, 16.6957) (6.4184, 16.7479) (6.4061, 16.787) (6.3979, 16.8131) (6.3937, 16.8262) knots 0 0 0 0 0 0 0.01428571 0.02857143 0.04285714 0.05714286 0.07142857 0.08571429 0.1 0.11428571 0.12857143 0.14285714 0.15714286 0.17142857 0.18571429 0.2 0.21428571 0.22857143 0.24285714 0.25714286 0.27142857 0.28571429 0.3 0.31428571 0.32857143 0.34285714 0.35714286 0.37142857 0.38571429 0.4 0.41428571 0.42857143 0.44285714 0.45714286 0.47142857 0.48571429 0.5 0.51428571 0.52857143 0.54285714 0.55714286 0.57142857 0.58571429 0.6 0.61428571 0.62857143 0.64285714 0.65714286 0.67142857 0.68571429 0.7 0.71428571 0.72857143 0.74285714 0.75714286 0.77142857 0.78571429 0.8 0.81428571 0.82857143 0.84285714 0.85714286 0.87142857 0.88571429 0.9 0.91428571 0.92857143 0.94285714 0.95714286 0.97142857 0.98571429 1 1 1 1 1 1
  arc A15 (6.3937, 16.8262) -> (4.7175, 17.3708) centre (0, 0) ccw
  spline S15 degree 5 poles (4.7175, 17.3708) (4.7065, 17.3627) (4.6845, 17.3464) (4.6516, 17.3219) (4.6079, 17.2892) (4.5536, 17.2479) (4.4997, 17.2065) (4.4462, 17.1647) (4.393, 17.1227) (4.3403, 17.0805) (4.2879, 17.038) (4.2358, 16.9952) (4.1842, 16.9523) (4.1329, 16.909) (4.0821, 16.8655) (4.0316, 16.8218) (3.9815, 16.7778) (3.9318, 16.7336) (3.8825, 16.6891) (3.8337, 16.6444) (3.7852, 16.5995) (3.7371, 16.5543) (3.6895, 16.5089) (3.6423, 16.4633) (3.5955, 16.4174) (3.5492, 16.3713) (3.5032, 16.3249) (3.4578, 16.2783) (3.4127, 16.2315) (3.3681, 16.1845) (3.324, 16.1372) (3.2803, 16.0897) (3.2371, 16.042) (3.1943, 15.994) (3.152, 15.9458) (3.1102, 15.8974) (3.0689, 15.8488) (3.028, 15.8) (2.9877, 15.7509) (2.9478, 15.7016) (2.9085, 15.6521) (2.8697, 15.6024) (2.8314, 15.5525) (2.7936, 15.5023) (2.7564, 15.452) (2.7197, 15.4014) (2.6836, 15.3506) (2.648, 15.2996) (2.613, 15.2484) (2.5785, 15.197) (2.5447, 15.1453) (2.5115, 15.0935) (2.4789, 15.0414) (2.447, 14.9891) (2.4158, 14.9366) (2.3853, 14.8839) (2.3553, 14.831) (2.3259, 14.7779) (2.2971, 14.7246) (2.2691, 14.6711) (2.2418, 14.6174) (2.2156, 14.5634) (2.1904, 14.5092) (2.1664, 14.4546) (2.1432, 14.3998) (2.1208, 14.3449) (2.099, 14.2898) (2.0776, 14.2346) (2.057, 14.1793) (2.0378, 14.1237) (2.0207, 14.0676) (2.0094, 14.0223) (2.0027, 13.9879) (1.9989, 13.9648) (1.9973, 13.9532) knots -1 -1 -1 -1 -1 -1 -0.98571429 -0.97142857 -0.95714286 -0.94285714 -0.92857143 -0.91428571 -0.9 -0.88571429 -0.87142857 -0.85714286 -0.84285714 -0.82857143 -0.81428571 -0.8 -0.78571429 -0.77142857 -0.75714286 -0.74285714 -0.72857143 -0.71428571 -0.7 -0.68571429 -0.67142857 -0.65714286 -0.64285714 -0.62857143 -0.61428571 -0.6 -0.58571429 -0.57142857 -0.55714286 -0.54285714 -0.52857143 -0.51428571 -0.5 -0.48571429 -0.47142857 -0.45714286 -0.44285714 -0.42857143 -0.41428571 -0.4 -0.38571429 -0.37142857 -0.35714286 -0.34285714 -0.32857143 -0.31428571 -0.3 -0.28571429 -0.27142857 -0.25714286 -0.24285714 -0.22857143 -0.21428571 -0.2 -0.18571429 -0.17142857 -0.15714286 -0.14285714 -0.12857143 -0.11428571 -0.1 -0.08571429 -0.07142857 -0.05714286 -0.04285714 -0.02857143 -0.01428571 0 0 0 0 0 0
  line L15 (1.9973, 13.9532) -> (1.6065, 11.2349)
  arc A16 (1.6065, 11.2349) -> (-1.6065, 11.2349) centre (0, 0) ccw
  line L16 (-1.6065, 11.2349) -> (-1.9973, 13.9532)
  spline S16 degree 5 poles (-1.9973, 13.9532) (-1.9989, 13.9648) (-2.0027, 13.9879) (-2.0094, 14.0223) (-2.0207, 14.0676) (-2.0378, 14.1237) (-2.057, 14.1793) (-2.0776, 14.2346) (-2.099, 14.2898) (-2.1208, 14.3449) (-2.1432, 14.3998) (-2.1664, 14.4546) (-2.1904, 14.5092) (-2.2156, 14.5634) (-2.2418, 14.6174) (-2.2691, 14.6711) (-2.2971, 14.7246) (-2.3259, 14.7779) (-2.3553, 14.831) (-2.3853, 14.8839) (-2.4158, 14.9366) (-2.447, 14.9891) (-2.4789, 15.0414) (-2.5115, 15.0935) (-2.5447, 15.1453) (-2.5785, 15.197) (-2.613, 15.2484) (-2.648, 15.2996) (-2.6836, 15.3506) (-2.7197, 15.4014) (-2.7564, 15.452) (-2.7936, 15.5023) (-2.8314, 15.5525) (-2.8697, 15.6024) (-2.9085, 15.6521) (-2.9478, 15.7016) (-2.9877, 15.7509) (-3.028, 15.8) (-3.0689, 15.8488) (-3.1102, 15.8974) (-3.152, 15.9458) (-3.1943, 15.994) (-3.2371, 16.042) (-3.2803, 16.0897) (-3.324, 16.1372) (-3.3681, 16.1845) (-3.4127, 16.2315) (-3.4578, 16.2783) (-3.5032, 16.3249) (-3.5492, 16.3713) (-3.5955, 16.4174) (-3.6423, 16.4633) (-3.6895, 16.5089) (-3.7371, 16.5543) (-3.7852, 16.5995) (-3.8337, 16.6444) (-3.8825, 16.6891) (-3.9318, 16.7336) (-3.9815, 16.7778) (-4.0316, 16.8218) (-4.0821, 16.8655) (-4.1329, 16.909) (-4.1842, 16.9523) (-4.2358, 16.9952) (-4.2879, 17.038) (-4.3403, 17.0805) (-4.393, 17.1227) (-4.4462, 17.1647) (-4.4997, 17.2065) (-4.5536, 17.2479) (-4.6079, 17.2892) (-4.6516, 17.3219) (-4.6845, 17.3464) (-4.7065, 17.3627) (-4.7175, 17.3708) knots 0 0 0 0 0 0 0.01428571 0.02857143 0.04285714 0.05714286 0.07142857 0.08571429 0.1 0.11428571 0.12857143 0.14285714 0.15714286 0.17142857 0.18571429 0.2 0.21428571 0.22857143 0.24285714 0.25714286 0.27142857 0.28571429 0.3 0.31428571 0.32857143 0.34285714 0.35714286 0.37142857 0.38571429 0.4 0.41428571 0.42857143 0.44285714 0.45714286 0.47142857 0.48571429 0.5 0.51428571 0.52857143 0.54285714 0.55714286 0.57142857 0.58571429 0.6 0.61428571 0.62857143 0.64285714 0.65714286 0.67142857 0.68571429 0.7 0.71428571 0.72857143 0.74285714 0.75714286 0.77142857 0.78571429 0.8 0.81428571 0.82857143 0.84285714 0.85714286 0.87142857 0.88571429 0.9 0.91428571 0.92857143 0.94285714 0.95714286 0.97142857 0.98571429 1 1 1 1 1 1
  arc A17 (-4.7175, 17.3708) -> (-6.3937, 16.8262) centre (0, 0) ccw
  spline S17 degree 5 poles (-6.3937, 16.8262) (-6.3979, 16.8131) (-6.4061, 16.787) (-6.4184, 16.7479) (-6.4345, 16.6957) (-6.4541, 16.6304) (-6.4734, 16.5652) (-6.4921, 16.5) (-6.5104, 16.4347) (-6.5283, 16.3695) (-6.5457, 16.3044) (-6.5627, 16.2392) (-6.5792, 16.1741) (-6.5953, 16.109) (-6.6109, 16.0439) (-6.626, 15.9788) (-6.6407, 15.9138) (-6.6549, 15.8488) (-6.6686, 15.7839) (-6.6819, 15.719) (-6.6947, 15.6542) (-6.707, 15.5894) (-6.7188, 15.5246) (-6.7302, 15.4599) (-6.7411, 15.3953) (-6.7515, 15.3308) (-6.7614, 15.2663) (-6.7708, 15.2019) (-6.7797, 15.1375) (-6.7881, 15.0732) (-6.7961, 15.009) (-6.8035, 14.9449) (-6.8104, 14.8809) (-6.8168, 14.817) (-6.8227, 14.7532) (-6.8281, 14.6894) (-6.8329, 14.6258) (-6.8373, 14.5623) (-6.8411, 14.4989) (-6.8443, 14.4356) (-6.8471, 14.3724) (-6.8493, 14.3094) (-6.8509, 14.2465) (-6.852, 14.1837) (-6.8524, 14.1211) (-6.8524, 14.0586) (-6.8518, 13.9963) (-6.8506, 13.9341) (-6.8488, 13.8721) (-6.8465, 13.8102) (-6.8435, 13.7486) (-6.8399, 13.6871) (-6.8356, 13.6258) (-6.8307, 13.5648) (-6.8251, 13.504) (-6.8188, 13.4433) (-6.812, 13.3829) (-6.8045, 13.3227) (-6.7965, 13.2627) (-6.7878, 13.2029) (-6.7782, 13.1435) (-6.7677, 13.0844) (-6.7562, 13.0257) (-6.7436, 12.9674) (-6.7301, 12.9095) (-6.7159, 12.8518) (-6.7012, 12.7944) (-6.6861, 12.7372) (-6.6702, 12.6804) (-6.6531, 12.6241) (-6.634, 12.5687) (-6.6164, 12.5253) (-6.6017, 12.4936) (-6.5911, 12.4727) (-6.5856, 12.4623) knots -1 -1 -1 -1 -1 -1 -0.98571429 -0.97142857 -0.95714286 -0.94285714 -0.92857143 -0.91428571 -0.9 -0.88571429 -0.87142857 -0.85714286 -0.84285714 -0.82857143 -0.81428571 -0.8 -0.78571429 -0.77142857 -0.75714286 -0.74285714 -0.72857143 -0.71428571 -0.7 -0.68571429 -0.67142857 -0.65714286 -0.64285714 -0.62857143 -0.61428571 -0.6 -0.58571429 -0.57142857 -0.55714286 -0.54285714 -0.52857143 -0.51428571 -0.5 -0.48571429 -0.47142857 -0.45714286 -0.44285714 -0.42857143 -0.41428571 -0.4 -0.38571429 -0.37142857 -0.35714286 -0.34285714 -0.32857143 -0.31428571 -0.3 -0.28571429 -0.27142857 -0.25714286 -0.24285714 -0.22857143 -0.21428571 -0.2 -0.18571429 -0.17142857 -0.15714286 -0.14285714 -0.12857143 -0.11428571 -0.1 -0.08571429 -0.07142857 -0.05714286 -0.04285714 -0.02857143 -0.01428571 0 0 0 0 0 0
  line L17 (-6.5856, 12.4623) -> (-5.3041, 10.0335)
  arc A18 (-5.3041, 10.0335) -> (-7.9034, 8.145) centre (0, 0) ccw
  line L18 (-7.9034, 8.145) -> (-9.8173, 10.1144)